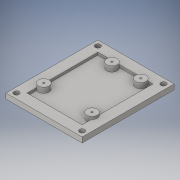
# Autodesk Inventor part: ArduinoMount
Saved by Autodesk Inventor 2016 (Build 200138000, 138)
## iProperties
Created: 2017-01-07
Part Number: ArduinoMount
Material: Generic
Document SubType Name: Modeling
Designer: james
Density: 1 g/cm^3
Appearance: Default
Author: james
Autodesk Inventor part; units mm, degrees
ref_plane "YZ Plane" through (0, 0, 0) normal (1, 0, 0) x (0, 1, 0)
ref_plane "XZ Plane" through (0, 0, 0) normal (0, 1, 0) x (-1, 0, 0)
ref_plane "XY Plane" through (0, 0, 0) normal (0, 0, 1) x (1, 0, 0)
sketch "Sketch1" plane through (0, 0, 0) normal (0, 1, 0) x (-1, 0, 0)
  line L0 (16.4526, 29.5814) -> (-36.8874, 29.5814)
  line L1 (-36.8874, 29.5814) -> (-36.8874, -38.9986)
  line L2 (-36.8874, -38.9986) -> (16.4526, -38.9986)
  line L3 (16.4526, -38.9986) -> (16.4526, 29.5814)
  point P0 (0, 0)
  dimension "d0" = 68.58
  dimension "d1" = 53.34
  constraints: 8 end point, 2 parallel, 1 horizontal, 1 perpendicular
  measures "d0" distance of L2.end L0.start
  measures "d1" distance of L0.start L0.end
extrude "Extrusion1" add sketch "Sketch1" along normal blind 2.54
sketch "Sketch2" plane through (0, 0, 0) normal (0, -1, 0) x (1, 0, 0)
  line L0 (-26.6126, -49.1586) -> (47.0474, -49.1586)
  line L1 (47.0474, -49.1586) -> (47.0474, 39.7414)
  line L2 (47.0474, 39.7414) -> (-26.6126, 39.7414)
  line L3 (-26.6126, 39.7414) -> (-26.6126, -49.1586)
  line L4 (-16.4526, -38.9986) -> (-16.4526, 29.5814) projected
  line L5 (36.8874, 29.5814) -> (36.8874, -38.9986) projected
  line L6 (-16.4526, 29.5814) -> (36.8874, 29.5814) projected
  line L7 (36.8874, -38.9986) -> (-16.4526, -38.9986) projected
  point P0 (0, 0)
  dimension "d4" = 10.16
  dimension "d5" = 10.16
  dimension "d6" = 10.16
  dimension "d7" = 10.16
  constraints: 8 end point, 2 parallel, 1 horizontal, 1 perpendicular
  measures "d4" distance between parallel lines of L3 L4
  measures "d5" distance between parallel lines of L5 L1
  measures "d6" distance between parallel lines of L2 L6
  measures "d7" distance between parallel lines of L7 L0
extrude "Extrusion2" add sketch "Sketch2" against normal blind 5.08
sketch "Sketch3" plane through (0, 5.08, 0) normal (0, 1, 0) x (1, 0, 0)
  line L0 (-26.6126, -39.7414) -> (47.0474, -39.7414) projected
  line L1 (-26.6126, 49.1586) -> (-26.6126, -39.7414) projected
  line L2 (47.0474, 49.1586) -> (-26.6126, 49.1586) projected
  line L3 (47.0474, -39.7414) -> (47.0474, 49.1586) projected
  point P0 (0, 0)
  point P1 (-21.5326, -34.6614)
  point P2 (41.9674, -34.6614)
  point P3 (41.9674, 44.0786)
  point P4 (-21.5326, 44.0786)
  dimension "d10" = 5.08
  dimension "d11" = 5.08
  dimension "d12" = 0
  dimension "d13" = 5.08
  dimension "d14" = 0
  dimension "d15" = 0
  dimension "d16" = 5.08
  dimension "d17" = 0
  measures "d10" distance from line of L0 point (-21.533, -34.661)
  measures "d11" distance from line of L1 point (-21.533, -34.661)
  measures "d12" horizontal distance of point (-21.533, 44.079) point (-21.533, -34.661)
  measures "d13" distance from line of L2 point (-21.533, 44.079)
  measures "d14" vertical distance of point (41.967, 44.079) point (-21.533, 44.079)
  measures "d15" vertical distance of point (-21.533, -34.661) point (41.967, -34.661)
  measures "d16" distance from line of L3 point (41.967, -34.661)
  measures "d17" horizontal distance of point (41.967, 44.079) point (41.967, -34.661)
hole "Hole1" at (-21.5326, 5.08, 34.6614) at (41.9674, 5.08, 34.6614) at (41.9674, 5.08, -44.0786) at (-21.5326, 5.08, -44.0786) direction (0, -1, 0) diameter 5.08 depth 25.4 tip angle 118
sketch "Sketch4" plane through (0, 2.54, 0) normal (0, 1, 0) x (1, 0, 0)
  circle A0 centre (-14.2126, -15.5814) radius 5.08
  circle A1 centre (33.5874, -16.6814) radius 5.08
  circle A2 centre (28.8874, 35.2186) radius 5.08
  circle A3 centre (0.9874, 35.2186) radius 5.08
  line L0 (36.8874, 38.9986) -> (36.8874, -29.5814) projected
  line L1 (-26.6126, -39.7414) -> (47.0474, -39.7414) projected
  line L2 (36.8874, -29.5814) -> (-16.4526, -29.5814) projected
  line L3 (-16.4526, -29.5814) -> (-16.4526, 38.9986) projected
  point P0 (0, 0)
  dimension "d25" = 10.16
  dimension "d26" = 10.16
  dimension "d27" = 10.16
  dimension "d28" = 10.16
  dimension "d36" = 27.9
  dimension "d41" = 51.9
  dimension "d42" = 50.8
  dimension "d43" = 15.2
  dimension "d44" = 0
  dimension "d45" = 3.3
  dimension "d46" = 4.7
  dimension "d47" = 14
  constraints: 4 centre point
  measures "d25" diameter of A0
  measures "d26" diameter of A1
  measures "d27" diameter of A2
  measures "d28" diameter of A3
  measures "d36" distance of A2.centre A3.centre
  measures "d41" vertical distance of A1.centre A2.centre
  measures "d42" vertical distance of A0.centre A3.centre
  measures "d43" horizontal distance of A3.centre A0.centre
  measures "d44" vertical distance of A2.centre A3.centre
  measures "d45" distance from line of A1.centre L0
  measures "d46" horizontal distance of A2.centre A1.centre
  measures "d47" distance from line of L2 A0.centre
extrude "Extrusion3" add sketch "Sketch4" along normal blind 5.08
sketch "Sketch5" plane through (0.9874, 7.62, -35.2186) normal (0, 1, 0) x (1, 0, 0)
  point P0 (-0.9874, -35.2186)
  point P1 (0, 0)
hole "Hole2" at (0.9874, 7.62, -35.2186) direction (0, -1, 0) diameter 1.778 depth 25.4 tip angle 118
sketch "Sketch6" plane through (28.8874, 7.62, -35.2186) normal (0, 1, 0) x (1, 0, 0)
  point P0 (-28.8874, -35.2186)
  point P1 (0, 0)
hole "Hole3" at (28.8874, 7.62, -35.2186) direction (0, -1, 0) diameter 1.778 depth 25.4 tip angle 118
sketch "Sketch7" plane through (33.5874, 7.62, 16.6814) normal (0, 1, 0) x (1, 0, 0)
  point P0 (-33.5874, 16.6814)
  point P1 (0, 0)
hole "Hole4" at (33.5874, 7.62, 16.6814) direction (0, -1, 0) diameter 1.778 depth 25.4 tip angle 118
sketch "Sketch8" plane through (-14.2126, 7.62, 15.5814) normal (0, 1, 0) x (1, 0, 0)
  point P0 (14.2126, 15.5814)
  point P1 (0, 0)
hole "Hole5" at (-14.2126, 7.62, 15.5814) direction (0, -1, 0) diameter 1.778 depth 25.4 tip angle 118
body "Solid1"
